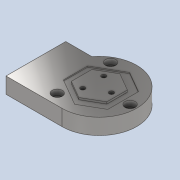
# Autodesk Inventor part: FFS080YS102U6
Saved by Autodesk Inventor 2022 (Build 260153000, 153)
## iProperties
Created: 2023-06-19
Part Number: FFS080YS102U6
Material: ステンレス鋼
Document SubType Name: Modeling
Designer: 81805
Density: 8 g/cm^3
Appearance: 半つや出し
Author: 81805
Autodesk Inventor part; units mm, degrees
ref_plane "YZ Plane" through (0, 0, 0) normal (1, 0, 0) x (0, 1, 0)
ref_plane "XZ Plane" through (0, 0, 0) normal (0, 1, 0) x (-1, 0, 0)
ref_plane "XY Plane" through (0, 0, 0) normal (0, 0, 1) x (1, 0, 0)
sketch "スケッチ1" plane through (0, 0, 0) normal (0, 0, 1) x (1, 0, 0)
  arc A0 (40, 0) -> (-24, -32) centre (0, 0) ccw
  line L0 (40, 0) -> (-24, 0)
  line L1 (-24, -32) -> (-24, -60)
  line L2 (-24, -60) -> (40, -60)
  line L3 (40, -60) -> (40, 0)
  circle A1 centre (0, 0) radius 33
  line L4 (-22, 0) -> (-11, 19.0526)
  line L5 (-11, 19.0526) -> (11, 19.0526)
  line L6 (11, 19.0526) -> (22, 0)
  line L7 (22, 0) -> (11, -19.0526)
  line L8 (11, -19.0526) -> (-11, -19.0526)
  line L9 (-11, -19.0526) -> (-22, 0)
  line L10 (-13, -25.5275) -> (13, -25.5275)
  line L11 (13, -25.5275) -> (29.4764, 3.0105)
  line L12 (29.4764, 3.0105) -> (16.4764, 25.5271)
  line L13 (16.4764, 25.5271) -> (-16.4764, 25.5271)
  line L14 (-16.4764, 25.5271) -> (-29.4764, 3.0105)
  line L15 (-29.4764, 3.0105) -> (-13, -25.5275)
  point P0 (-24, -32)
  point P1 (0, 33)
  point P2 (-28.5788, -16.5)
  point P3 (28.5788, -16.5)
  dimension "d34" = 66
  dimension "d0" = 80
  dimension "d1" = 0
  dimension "d2" = 64
  dimension "d3" = 60
  dimension "d35" = 0
  dimension "d38" = 360
  dimension "d62" = 22
  dimension "d94" = 0
  dimension "d95" = 26
  dimension "d96" = 120
  dimension "d97" = 26
  dimension "d98" = 120
  dimension "d99" = 120
  dimension "d100" = 26
  dimension "d101" = 120
  dimension "d102" = 13
  dimension "d103" = 25.5275
  constraints: 32 end point, 4 parallel, 2 coincident, 2 horizontal, 2 point on circle, 1 centre point, 1 perpendicular, 1 point on line, 1 vertical alignment, 19 other
  measures "d0" diameter of A0
  measures "d1" distance from line of L0 point (0, 0)
  measures "d2" distance of L1.end L2.end
  measures "d3" distance from line of A0.centre L2
  measures "d35" horizontal distance of point (0, 0) point (0, 33)
  measures "d62" distance of L7.end L8.end
  measures "d94" distance of point (0, 0) point (0, 0)
  measures "d95" distance of L10.start L10.end
  measures "d96" angle of L11 L10
  measures "d97" distance of L11.end L12.end
  measures "d98" angle of L12 L11
  measures "d99" angle of L13 L12
  measures "d100" distance of L13.end L14.end
  measures "d101" angle of L14 L13
  measures "d102" horizontal distance of point (0, 0) L10.start
  measures "d103" distance from line of point (0, 0) L10
extrude "押し出し1" add sketch "スケッチ1" against normal blind 17 contours L3 L2 L1 A0 | L7 L8 L9 L0 | L0 L4 L5 L6 | L11 L10 L15 L14 L13 L12 | A1
hole "穴3" at (0, 33, 0) at (-28.5788, -16.5, 0) at (28.5788, -16.5, 0) direction (0, 0, -1) diameter 6.4 depth 17 tip angle 118 counterbore diameter 11 counterbore depth 6
sketch "スケッチ2" plane through (0, 0, -17) normal (0, 0, -1) x (-1, 0, 0)
  circle A0 centre (0, 0) radius 35
  point P0 (-35, 0)
  point P1 (35, 0)
  dimension "d47" = 70
  dimension "d48" = 0
  dimension "d51" = 360
  constraints: 1 coincident, 1 horizontal alignment, 5 other
  measures "d48" vertical distance of point (0, 0) point (-35, 0)
hole "穴4" at (35, 0, -17) at (-35, 0, -17) direction (0, 0, 1) diameter 4 depth 4 tip angle 118
extrude "押し出し2" add sketch "スケッチ1" along normal blind 1 contours L7 L8 L9 L0 | L0 L4 L5 L6
sketch "スケッチ4" plane through (0, 0, 1) normal (0, 0, 1) x (1, 0, 0)
  circle A0 centre (0, 0) radius 13
  point P0 (0, 13)
  point P1 (-11.2583, -6.5)
  point P2 (11.2583, -6.5)
  dimension "d81" = 26
  dimension "d82" = 0
  dimension "d85" = 360
  constraints: 1 coincident, 1 vertical alignment, 6 other
  measures "d82" horizontal distance of point (0, 0) point (0, 13)
hole "穴5" at (0, 13, 1) at (-11.2583, -6.5, 1) at (11.2583, -6.5, 1) direction (0, 0, -1) diameter 4.917 depth 10 tip angle 118 thread size "M6x1" designation "M6" class "6H" standard "GB Metric profile"
extrude "押し出し3" cut sketch "スケッチ1" against normal blind 1 contours L11 L10 L15 L14 L13 L12
